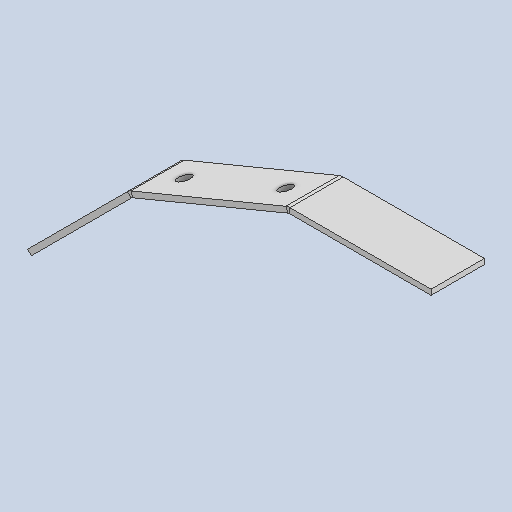
# Autodesk Inventor part: ДМФ 01 52 Верхний лист
Saved by Autodesk Inventor 2024.2 (Build 282272000, 272)
## iProperties
Created: 2024-05-05
Part Number: ДМФ 01 52 Верхний лист
Material: Generic
Document SubType Name: Sheet Metal
Designer: pokla
Density: 1 g/cm^3
Sheet Metal Rule: Default
Appearance: Default
Author: pokla
Autodesk Inventor part; units mm, degrees
note: some values were not read from the file. Chosen so that the rebuilt part matches the saved one: flange form of "Plate1".
ref_plane "YZ Plane" through (0, 0, 0) normal (1, 0, 0) x (0, 1, 0)
ref_plane "XZ Plane" through (0, 0, 0) normal (0, 1, 0) x (-1, 0, 0)
ref_plane "XY Plane" through (0, 0, 0) normal (0, 0, 1) x (1, 0, 0)
sketch "Sketch2" plane through (0, 0, 0) normal (0, 0, 1) x (1, 0, 0)
  line L0 (0, 277.6336) -> (196.3166, 196.3166) construction
  line L1 (196.3166, 196.3166) -> (277.6336, 0) construction
  line L2 (277.6336, 0) -> (196.3166, -196.3166) construction
  line L3 (196.3166, -196.3166) -> (0, -277.6336) construction
  line L4 (0, -277.6336) -> (-196.3166, -196.3166) construction
  line L5 (-196.3166, -196.3166) -> (-277.6336, 0) construction
  line L6 (-277.6336, 0) -> (-196.3166, 196.3166) construction
  line L7 (-196.3166, 196.3166) -> (0, 277.6336) construction
  line L8 (-196.3166, 196.3166) -> (0, 277.6336) construction
  line L9 (-461.2666, 773.8898) -> (-221.0579, 873.3874) construction
  line L10 (-98.1583, 236.9751) -> (-341.1623, 823.6386) construction
  line L11 (-221.0579, 873.3874) -> (0, 873.3874) construction
  line L12 (0, 873.3874) -> (0, 277.6336) construction
  line L13 (-461.2666, 773.8898) -> (-617.5782, 617.5782) construction
  line L14 (-617.5782, 617.5782) -> (-196.3166, 196.3166) construction
  line L15 (-223.0037, 867.1695) -> (-339.2489, 819.0192)
  line L16 (-5, 868.3874) -> (-216.8808, 868.3874)
  line L17 (-455.494, 770.8689) -> (-339.2489, 819.0192)
  line L18 (-610.5071, 617.5782) -> (-460.6848, 767.4005)
  arc A0 (-216.8808, 868.3874) -> (-223.0037, 867.1695) centre (-216.8808, 852.3874) ccw
  arc A1 (-455.494, 770.8689) -> (-460.6848, 767.4005) centre (-449.3711, 756.0868) ccw
  point P0 (0, 0)
  point P1 (0, 0)
  point P2 (0, 0)
  point P3 (-220.0634, 868.3874)
  point P4 (-458.4343, 769.651)
  dimension "d0" = 513
  dimension "d1" = 260
  dimension "d2" = 635
  dimension "d6" = 5
  dimension "d10" = 5
  dimension "d14" = 5
  dimension "d15" = 16
  measures "d0" distance between parallel lines of L5 L1
  measures "d1" distance of L13.start L11.start
  measures "d2" distance of L10.end L10.start
  measures "d6" distance between parallel lines of L9 L15
  measures "d10" distance between parallel lines of L11 L16
  measures "d14" distance from line of L12 L16.start
  measures "d15" radius of A0
contour flange "Contour Flange1" sketch "Sketch2" thickness 8 bend radius 8 width 80 along (0, 0, 1) mid plane no both sides no wall seen from (-110.9404, 868.3874, 0) lies toward (0, -1, 0) curves L16 A0 L15 L17 A1 L18
bend "Bend1"
corner "Corner1"
sketch "Sketch3" plane through (-455.494, 770.8689, 80) normal (-0.3826834, 0.9238795, 0) x (0.9238795, 0.3826834, 0)
  line L0 (125.8228, 80) -> (125.8228, 0) construction
  line L1 (0, 0) -> (251.6457, 0) projected
  circle A0 centre (43.3228, 40) radius 10
  circle A1 centre (208.3228, 40) radius 10
  point P0 (125.8228, 40)
  dimension "d27" = 20
  dimension "d28" = 82.5
  constraints: 2 centre point, 2 end point, 2 horizontal alignment, 2 midpoint, 1 equal radius, 1 other
  measures "d27" diameter of A0
  measures "d28" distance of A0.centre point (125.823, 40)
extrude "Extrusion1" cut sketch "Sketch3" against normal up to surface (8 mm away)
equation "\"d0\" = Барабан_габарит_по_кассетам"
equation "\"d1\" = Кассета_длина_грани"
equation "\"d2\" = Кассета_высота"
equation "\"d10\" = d6"
equation "\"d15\" = BendRadius + Thickness"
equation "\"d16\" = Thickness"
equation "\"d17\" = BendReliefWidth"
equation "\"d18\" = BendReliefDepth"
equation "\"d19\" = MinimumRemnant"
equation "\"d20\" = TransitionRadius"
equation "\"d22\" = BendRadius"
equation "\"d24\" = CornerReliefSize"
equation "\"d25\" = GapSize"
equation "\"d26\" = JacobiRadiusSize"
equation "\"BendRadius\" = Thickness"
equation "\"BendReliefWidth\" = Thickness"
equation "\"BendReliefDepth\" = 0.5 * Thickness"
equation "\"CornerReliefSize\" = 4 * Thickness"
equation "\"MinimumRemnant\" = 2 * Thickness"
equation "\"TransitionRadius\" = BendRadius"
equation "\"JacobiRadiusSize\" = BendRadius"
equation "\"GapSize\" = Thickness"
equation "\"Барабан_габарит_по_кассетам\" = 513"
equation "\"Кассета_длина_грани\" = 260"
equation "\"Кассета_высота\" = 635"
equation "\"Thickness\" = 8"
body "Solid1"
